LRS-600-36 (Autodesk Fusion 360 design; units mm, degrees)
Autodesk Fusion 360 part; units mm, degrees
sketch "Sketch1" plane through (0, 0, 0) normal (0, 0, 1) x (1, 0, 0)
  line L0 (62, 112.5) -> (-62, 112.5)
  line L1 (-62, 112.5) -> (-62, -112.5)
  line L2 (-62, -112.5) -> (62, -112.5)
  line L3 (62, -112.5) -> (62, 112.5)
  line L4 (62, 112.5) -> (-62, -112.5) construction
  line L5 (-62, 112.5) -> (62, -112.5) construction
  dimension "d1" = 124
  dimension "d2" = 225
  constraint horizontal L0
  constraint perpendicular L0 L1
  constraint parallel L0 L2
  constraint parallel L1 L3
  constraint coincident L4 origin
  constraint coincident L5 origin
  measures "d1" distance of L1.end L2.end
  measures "d2" distance of L0.end L1.end
extrude "Extrude1" add sketch "Sketch1" along normal blind 41 makes body 1
sketch "Sketch2" plane through (62, 0, 0) normal (1, 0, 0) x (0, 1, 0)
  line L0 (-112.5, 0) -> (112.5, 0)
  line L1 (112.5, 0) -> (112.5, 41)
  line L2 (112.5, 41) -> (-112.5, 41)
  line L3 (-112.5, 41) -> (-112.5, 0)
  circle A0 centre (-85.8, 31) radius 2
  circle A1 centre (-85.8, 13) radius 2
  circle A2 centre (74.2, 31) radius 2
  circle A3 centre (74.2, 13) radius 2
  line L4 (-85.8, 0) -> (-85.8, 41) construction
  line L5 (74.2, 0) -> (74.2, 41) construction
  line L6 (-85.8, 31) -> (74.2, 31) construction
  line L7 (-85.8, 13) -> (74.2, 13) construction
  dimension "d5" = 4
  dimension "d6" = 26.7
  dimension "d7" = 160
  dimension "d8" = 13
  dimension "d9" = 18
  constraint equal A0 A1
  constraint equal A1 A2
  constraint equal A2 A3
  constraint coincident L0 L4.start
  constraint coincident L2 L4.end
  constraint perpendicular L2 L4
  constraint coincident L0 L5.start
  constraint coincident L2 L5.end
  constraint perpendicular L2 L5
  constraint coincident A0.centre L4
  constraint coincident A1.centre L4
  constraint coincident A2.centre L5
  constraint coincident A3.centre L5
  constraint coincident A0.centre L6.start
  constraint coincident L5 A2.centre
  constraint perpendicular L5 L6
  constraint coincident A1.centre L7.start
  constraint coincident L5 A3.centre
  constraint perpendicular L5 L7
  constraint coincident A2.centre L6
  constraint coincident A3.centre L7
  measures "d5" diameter of A0
  measures "d6" distance of L3 L4
  measures "d7" distance of L4 L5
  measures "d8" distance of A1.centre L4.start
  measures "d9" distance of A0.centre A1.centre
shell "Shell1" thickness 2 removed faces 0 bodies 1
extrude "Extrude2" cut sketch "Sketch2" against normal through all contours A0 | A1 | A2 | A3 bodies 1
sketch "Sketch3" plane through (0, 0, 41) normal (0, 0, 1) x (-1, 0, 0)
  line L0 (-62, 112.5) -> (-62, -112.5)
  line L1 (-62, -112.5) -> (62, -112.5)
  line L2 (62, -112.5) -> (62, 112.5)
  line L3 (62, 112.5) -> (-62, 112.5)
  line L4 (62, 96.1) -> (-62, 96.1)
  line L5 (-60, 112.5) -> (-60, 96.1)
  line L6 (60, 96.1) -> (60, 112.5)
  dimension "d12" = 16.4
  constraint coincident L2 L4.start
  constraint coincident L0 L4.end
  constraint perpendicular L0 L4
  constraint coincident L4 L6.start
  constraint coincident L4 L5.end
  measures "d12" distance of L3 L4
extrude "Extrude3" cut sketch "Sketch3" against normal up to surface (39 mm away) contours L3 L4 L5 L6 bodies 1
sketch "Sketch4" plane through (0, 0, 0) normal (0, 0, -1) x (1, 0, 0)
  line L0 (62, -112.5) -> (62, 112.5)
  line L1 (62, 112.5) -> (-62, 112.5)
  line L2 (-62, 112.5) -> (-62, -112.5)
  line L3 (-62, -112.5) -> (62, -112.5)
  line L4 (25.5, 79) -> (-24.5, 79) construction
  line L5 (-24.5, 79) -> (-24.5, -71) construction
  line L6 (-24.5, -71) -> (25.5, -71) construction
  line L7 (25.5, -71) -> (25.5, 79) construction
  circle A0 centre (-24.5, 79) radius 2
  circle A1 centre (25.5, 79) radius 2
  circle A2 centre (25.5, -71) radius 2
  circle A3 centre (-24.5, -71) radius 2
  dimension "d18" = 150
  dimension "d19" = 50
  dimension "d21" = 33.5
  dimension "d22" = 37.5
  dimension "d23" = 4
  constraint horizontal L4
  constraint vertical L5
  constraint horizontal L6
  constraint vertical L7
  constraint coincident L4.end L5.start
  constraint coincident L4.start L7.end
  constraint coincident L6.end L7.start
  constraint coincident L5.end L6.start
  constraint equal A0 A1
  constraint equal A1 A2
  constraint equal A2 A3
  measures "d18" distance of L4.start L6.end
  measures "d19" distance of L4.start L4.end
  measures "d21" distance of L1 L4
  measures "d22" distance of L2 L5
  measures "d23" diameter of A0
extrude "Extrude4" cut sketch "Sketch4" against normal blind 2 contours A0 | A1 | A2 | A3 bodies 1
sketch "Sketch5" plane through (0, 0, 2) normal (0, 0, 1) x (-1, 0, 0)
  circle A0 centre (24.5, 79) radius 2
  circle A1 centre (-25.5, -71) radius 2
  circle A2 centre (-25.5, 79) radius 2
  circle A3 centre (24.5, -71) radius 2
  line L0 (-60, 112.5) -> (-60, -110.5)
  line L1 (-60, -110.5) -> (60, -110.5)
  line L2 (60, -110.5) -> (60, 112.5)
  line L3 (60, 112.5) -> (-60, 112.5)
extrude "Extrude5" add sketch "Sketch5" along normal blind 1.7 from surface at 3 separate body contours A0 | A1 | A2 | A3 | L0 L1 L2 L3 makes body 2
sketch "Sketch6" plane through (0, 0, 6.7) normal (0, 0, 1) x (-1, 0, 0)
  line L0 (60, 112.5) -> (-60, 112.5)
  line L1 (-60, 112.5) -> (-60, -110.5)
  line L2 (-60, -110.5) -> (60, -110.5)
  line L3 (60, -110.5) -> (60, 112.5)
  line L4 (-52.7, 110.9) -> (34.3, 110.9)
  line L5 (34.3, 110.9) -> (34.3, 92.9)
  line L6 (34.3, 92.9) -> (-52.7, 92.9)
  line L7 (-52.7, 92.9) -> (-52.7, 110.9)
  dimension "d29" = 87
  dimension "d30" = 18
  dimension "d31" = 1.6
  dimension "d32" = 7.3
  constraint horizontal L4
  constraint vertical L5
  constraint horizontal L6
  constraint vertical L7
  measures "d29" distance of L4.start L4.end
  measures "d30" distance of L4.start L6.end
  measures "d31" distance of L0 L4
  measures "d32" distance of L1 L7
extrude "Extrude6" add sketch "Sketch6" along normal blind 15.4 separate body contours L4 L5 L6 L7 makes body 3
sketch "Sketch7" plane through (0, 0, 6.7) normal (0, 0, 1) x (-1, 0, 0)
  line L0 (60, 112.5) -> (-60, 112.5)
  line L1 (-60, 112.5) -> (-60, -110.5)
  line L2 (-60, -110.5) -> (60, -110.5)
  line L3 (60, -110.5) -> (60, 112.5)
  circle A0 centre (44, 106) radius 3.5
  circle A1 centre (53.5, 107) radius 1.5
  dimension "d35" = 3
  dimension "d36" = 7
  dimension "d37" = 6.5
  dimension "d38" = 5.5
  dimension "d39" = 6.5
  dimension "d40" = 16
  measures "d35" diameter of A1
  measures "d36" diameter of A0
  measures "d37" distance of L3 A1.centre
  measures "d38" distance of L0 A1.centre
  measures "d39" distance of L0 A0.centre
  measures "d40" distance of L3 A0.centre
extrude "Extrude7" add sketch "Sketch7" along normal blind 10 contours A1 bodies 2
extrude "Extrude8" add sketch "Sketch7" along normal blind 8 contours A0 bodies 2
sketch "Sketch8" plane through (0, 0, 22.1) normal (0, 0, 1) x (-1, 0, 0)
  line L0 (-52.7, 92.9) -> (34.3, 92.9)
  line L1 (34.3, 92.9) -> (34.3, 110.9)
  line L2 (34.3, 110.9) -> (-52.7, 110.9)
  line L3 (-52.7, 110.9) -> (-52.7, 92.9)
  line L4 (-52.7, 110.9) -> (-51.5, 110.9)
  line L5 (-51.5, 110.9) -> (-51.5, 95.9)
  line L6 (-51.5, 95.9) -> (-43.3, 95.9)
  line L7 (-43.3, 95.9) -> (-43.3, 110.9)
  line L8 (-41.95, 110.9) -> (-41.95, 95.9)
  line L9 (-41.95, 95.9) -> (-33.75, 95.9)
  line L10 (-33.75, 95.9) -> (-33.75, 110.9)
  line L11 (-32.4, 110.9) -> (-32.4, 95.9)
  line L12 (-32.4, 95.9) -> (-24.2, 95.9)
  line L13 (-24.2, 95.9) -> (-24.2, 110.9)
  line L14 (-22.85, 110.9) -> (-22.85, 95.9)
  line L15 (-22.85, 95.9) -> (-14.65, 95.9)
  line L16 (-14.65, 95.9) -> (-14.65, 110.9)
  line L17 (-13.3, 110.9) -> (-13.3, 95.9)
  line L18 (-13.3, 95.9) -> (-5.1, 95.9)
  line L19 (-5.1, 95.9) -> (-5.1, 110.9)
  line L20 (-3.75, 110.9) -> (-3.75, 95.9)
  line L21 (-3.75, 95.9) -> (4.45, 95.9)
  line L22 (4.45, 95.9) -> (4.45, 110.9)
  line L23 (5.8, 110.9) -> (5.8, 95.9)
  line L24 (5.8, 95.9) -> (14, 95.9)
  line L25 (14, 95.9) -> (14, 110.9)
  line L26 (15.35, 110.9) -> (15.35, 95.9)
  line L27 (15.35, 95.9) -> (23.55, 95.9)
  line L28 (23.55, 95.9) -> (23.55, 110.9)
  line L29 (24.9, 110.9) -> (24.9, 95.9)
  line L30 (24.9, 95.9) -> (33.1, 95.9)
  line L31 (33.1, 95.9) -> (33.1, 110.9)
  line L32 (24.9, 110.9) -> (23.55, 110.9)
  line L33 (15.35, 110.9) -> (14, 110.9)
  line L34 (5.8, 110.9) -> (4.45, 110.9)
  line L35 (-3.75, 110.9) -> (-5.1, 110.9)
  line L36 (-13.3, 110.9) -> (-14.65, 110.9)
  line L37 (-22.85, 110.9) -> (-24.2, 110.9)
  line L38 (-32.4, 110.9) -> (-33.75, 110.9)
  line L39 (-41.95, 110.9) -> (-43.3, 110.9)
  line L40 (34.3, 110.9) -> (33.1, 110.9)
  dimension "d45" = 8.2
  dimension "d46" = 1.35
  dimension "d47" = 15
  constraint coincident L2.end L3.start
  constraint coincident L2 L4.end
  constraint perpendicular L3 L4
  constraint perpendicular L4 L5
  constraint perpendicular L3 L6
  constraint coincident L2 L7.end
  constraint perpendicular L4 L7
  constraint perpendicular L4 L8
  constraint perpendicular L7 L9
  constraint coincident L2 L10.end
  constraint perpendicular L2 L10
  constraint coincident L2 L11.start
  constraint perpendicular L2 L11
  constraint perpendicular L11 L12
  constraint coincident L2 L13.end
  constraint perpendicular L2 L13
  constraint coincident L2 L14.start
  constraint perpendicular L2 L14
  constraint perpendicular L14 L15
  constraint coincident L2 L16.end
  constraint perpendicular L2 L16
  constraint coincident L2 L17.start
  constraint perpendicular L2 L17
  constraint perpendicular L17 L18
  constraint coincident L2 L19.end
  constraint perpendicular L2 L19
  constraint coincident L2 L20.start
  constraint perpendicular L2 L20
  constraint perpendicular L19 L21
  constraint coincident L2 L22.end
  constraint perpendicular L21 L22
  constraint coincident L2 L23.start
  constraint perpendicular L2 L23
  constraint perpendicular L19 L24
  constraint coincident L2 L25.end
  constraint perpendicular L2 L25
  constraint coincident L2 L26.start
  constraint perpendicular L2 L26
  constraint perpendicular L26 L27
  constraint coincident L2 L28.end
  constraint perpendicular L2 L28
  constraint coincident L2 L29.start
  constraint perpendicular L2 L29
  constraint perpendicular L29 L30
  constraint coincident L2 L31.end
  constraint perpendicular L2 L31
  constraint equal L27 L30
  constraint equal L24 L27
  constraint equal L21 L24
  constraint equal L18 L21
  constraint equal L15 L18
  constraint equal L12 L15
  constraint equal L9 L12
  constraint equal L6 L9
  constraint perpendicular L8 L39
  constraint equal L38 L39
  constraint equal L37 L38
  constraint equal L36 L37
  constraint equal L35 L36
  constraint equal L34 L35
  constraint equal L33 L34
  constraint equal L32 L33
  constraint coincident L1.end L2.start
  constraint equal L4 L40
  constraint collinear L27 L30
  constraint collinear L24 L27
  constraint collinear L21 L24
  constraint collinear L15 L21
  constraint collinear L15 L18
  constraint collinear L12 L18
  constraint collinear L9 L12
  constraint collinear L6 L9
  measures "d45" distance of L29.end L30.end
  measures "d46" distance of L7.end L8.start
  measures "d47" distance of L4.end L5.end
extrude "Extrude9" cut sketch "Sketch8" against normal blind 8 contours L2 L5 L6 L7 | L2 L29 L30 L31 | L2 L8 L9 L10 | L2 L26 L27 L28 | L2 L11 L12 L13 | L2 L23 L24 L25 | L2 L14 L15 L16 | L2 L20 L21 L22 | L2 L17 L18 L19 bodies 3
sketch "Sketch9" plane through (0, 0, 41) normal (0, 0, 1) x (-1, 0, 0)
  line L0 (-60, 96.1) -> (-60, 112.5)
  line L1 (-60, 112.5) -> (-62, 112.5)
  line L2 (-62, 112.5) -> (-62, -112.5)
  line L3 (-62, -112.5) -> (62, -112.5)
  line L4 (62, -112.5) -> (62, 112.5)
  line L5 (62, 112.5) -> (60, 112.5)
  line L6 (60, 112.5) -> (60, 96.1)
  line L7 (60, 96.1) -> (-60, 96.1)
  circle A0 centre (24.5, -62.5) radius 30 construction
  circle A1 centre (24.5, -62.5) radius 26.5 construction
  circle A2 centre (24.5, -62.5) radius 18.5 construction
  circle A3 centre (24.5, -62.5) radius 21.5
  circle A4 centre (24.5, -62.5) radius 15.5
  circle A5 centre (24.5, -62.5) radius 29.5
  circle A6 centre (24.5, -62.5) radius 23.5
  line L8 (24.5, -62.5) -> (62, -62.5) construction
  line L9 (24.5, -62.5) -> (62, -72.5481) construction
  circle A7 centre (42.3696, -67.2882) radius 3
  circle A8 centre (42.3696, -57.7118) radius 3
  circle A9 centre (37.5815, -49.4185) radius 3
  circle A10 centre (29.2882, -44.6304) radius 3
  circle A11 centre (19.7118, -44.6304) radius 3
  circle A12 centre (11.4185, -49.4185) radius 3
  circle A13 centre (6.6304, -57.7118) radius 3
  circle A14 centre (6.6304, -67.2882) radius 3
  circle A15 centre (11.4185, -75.5815) radius 3
  circle A16 centre (19.7118, -80.3696) radius 3
  circle A17 centre (29.2882, -80.3696) radius 3
  circle A18 centre (37.5815, -75.5815) radius 3
  line L10 (24.5, -62.5) -> (25.2686, -62.7059) construction
  line L11 (24.5, -62.5) -> (62, -69.1123) construction
  circle A19 centre (50.5974, -67.1017) radius 3
  circle A20 centre (50.5974, -57.8983) radius 3
  circle A21 centre (47.4497, -49.25) radius 3
  circle A22 centre (41.5339, -42.1998) radius 3
  circle A23 centre (33.5635, -37.5981) radius 3
  circle A24 centre (24.5, -36) radius 3
  circle A25 centre (15.4365, -37.5981) radius 3
  circle A26 centre (7.4661, -42.1998) radius 3
  circle A27 centre (1.5503, -49.25) radius 3
  circle A28 centre (-1.5974, -57.8983) radius 3
  circle A29 centre (-1.5974, -67.1017) radius 3
  circle A30 centre (1.5503, -75.75) radius 3
  circle A31 centre (7.4661, -82.8002) radius 3
  circle A32 centre (15.4365, -87.4019) radius 3
  circle A33 centre (24.5, -89) radius 3
  circle A34 centre (33.5635, -87.4019) radius 3
  circle A35 centre (41.5339, -82.8002) radius 3
  circle A36 centre (47.4497, -75.75) radius 3
  dimension "d50" = 37.5
  dimension "d51" = 50
  dimension "d52" = 60
  dimension "d53" = 53
  dimension "d54" = 37
  dimension "d55" = 3
  dimension "d56" = -3
  dimension "d57" = 3
  dimension "d58" = -3
  dimension "d59" = 15
  dimension "d61" = 360
  dimension "d62" = 10
  dimension "d64" = 360
  constraint concentric A0 A1
  constraint concentric A0 A2
  constraint coincident A0.centre A1.centre
  constraint perpendicular L4 L8
  constraint coincident L4 L9.end
  constraint coincident L4 L8.end
  constraint coincident A2 A7.centre
  constraint coincident L9 A7.centre
  constraint tangent A4 A7
  constraint coincident L9 L10.end
  constraint coincident L4 L11.end
  constraint coincident A1 A19.centre
  constraint coincident L11 A19.centre
  constraint tangent A6 A19
  measures "d50" distance of L4 A0.centre
  measures "d51" distance of L3 A0.centre
  measures "d52" diameter of A0
  measures "d53" diameter of A1
  measures "d54" diameter of A2
  measures "d59" angle of L8 L9
  measures "d62" angle of L8 L11
extrude "Extrude10" cut sketch "Sketch9" against normal blind 2 contours A3 A4 A7 A8 | A8 | A7 | A3 A4 A9 A10 | A9 | A3 A4 A17 A18 | A18 | A10 | A17 | A3 A4 A11 A12 | A11 | A3 A4 A15 A16 | A16 | A12 | A15 | A3 A4 A13 A14 | A13 | A14 | A5 A6 A20 A21 | A20 | A5 A6 A19 A36 | A19 | A5 A6 A21 A22 | A21 | A5 A6 A35 A36 | A36 | A22 | A35 | A5 A6 A23 A24 | A23 | A5 A6 A33 A34 | A34 | A5 A6 A24 A25 | A24 | A5 A6 A32 A33 | A33 | A25 | A32 | A5 A6 A26 A27 | A26 | A5 A6 A30 A31 | A31 | A5 A6 A27 A28 | A27 | A5 A6 A29 A30 | A30 | A28 | A29 bodies 1
sketch "Sketch10" plane through (0, 0, 41) normal (0, 0, 1) x (-1, 0, 0)
  arc A0 (14.4104, -90.2209) -> (34.5896, -90.2209) centre (24.5, -62.5) ccw
  arc A1 (16.4625, -84.5828) -> (14.4104, -90.2209) centre (15.4365, -87.4019) ccw
  arc A2 (16.4625, -84.5828) -> (32.5375, -84.5828) centre (24.5, -62.5) ccw
  arc A3 (34.5896, -90.2209) -> (32.5375, -84.5828) centre (33.5635, -87.4019) ccw
  arc A4 (18.9354, -41.7326) -> (9.2972, -47.2972) centre (24.5, -62.5) ccw
  arc A5 (20.4883, -47.5281) -> (18.9354, -41.7326) centre (19.7118, -44.6304) ccw
  arc A6 (20.4883, -47.5281) -> (13.5398, -51.5398) centre (24.5, -62.5) ccw
  arc A7 (9.2972, -47.2972) -> (13.5398, -51.5398) centre (11.4185, -49.4185) ccw
  arc A8 (45.2674, -68.0646) -> (45.2674, -56.9354) centre (24.5, -62.5) ccw
  arc A9 (39.4719, -66.5117) -> (45.2674, -68.0646) centre (42.3696, -67.2882) ccw
  arc A10 (39.4719, -66.5117) -> (39.4719, -58.4883) centre (24.5, -62.5) ccw
  arc A11 (45.2674, -56.9354) -> (39.4719, -58.4883) centre (42.3696, -57.7118) ccw
  arc A12 (30.0646, -83.2674) -> (39.7028, -77.7028) centre (24.5, -62.5) ccw
  arc A13 (28.5117, -77.4719) -> (30.0646, -83.2674) centre (29.2882, -80.3696) ccw
  arc A14 (28.5117, -77.4719) -> (35.4602, -73.4602) centre (24.5, -62.5) ccw
  arc A15 (39.7028, -77.7028) -> (35.4602, -73.4602) centre (37.5815, -75.5815) ccw
  arc A16 (34.5896, -34.7791) -> (14.4104, -34.7791) centre (24.5, -62.5) ccw
  arc A17 (32.5375, -40.4172) -> (34.5896, -34.7791) centre (33.5635, -37.5981) ccw
  arc A18 (32.5375, -40.4172) -> (16.4625, -40.4172) centre (24.5, -62.5) ccw
  arc A19 (14.4104, -34.7791) -> (16.4625, -40.4172) centre (15.4365, -37.5981) ccw
  arc A20 (43.4622, -85.0983) -> (53.5518, -67.6226) centre (24.5, -62.5) ccw
  arc A21 (39.6055, -80.502) -> (43.4622, -85.0983) centre (41.5339, -82.8002) ccw
  arc A22 (39.6055, -80.502) -> (47.643, -66.5807) centre (24.5, -62.5) ccw
  arc A23 (53.5518, -67.6226) -> (47.643, -66.5807) centre (50.5974, -67.1017) ccw
  arc A24 (-4.5518, -67.6226) -> (5.5378, -85.0983) centre (24.5, -62.5) ccw
  arc A25 (1.357, -66.5807) -> (-4.5518, -67.6226) centre (-1.5974, -67.1017) ccw
  arc A26 (1.357, -66.5807) -> (9.3945, -80.502) centre (24.5, -62.5) ccw
  arc A27 (5.5378, -85.0983) -> (9.3945, -80.502) centre (7.4661, -82.8002) ccw
  arc A28 (3.7326, -56.9354) -> (3.7326, -68.0646) centre (24.5, -62.5) ccw
  arc A29 (9.5281, -58.4883) -> (3.7326, -56.9354) centre (6.6304, -57.7118) ccw
  arc A30 (9.5281, -58.4883) -> (9.5281, -66.5117) centre (24.5, -62.5) ccw
  arc A31 (3.7326, -68.0646) -> (9.5281, -66.5117) centre (6.6304, -67.2882) ccw
  arc A32 (39.7028, -47.2972) -> (30.0646, -41.7326) centre (24.5, -62.5) ccw
  arc A33 (35.4602, -51.5398) -> (39.7028, -47.2972) centre (37.5815, -49.4185) ccw
  arc A34 (35.4602, -51.5398) -> (28.5117, -47.5281) centre (24.5, -62.5) ccw
  arc A35 (30.0646, -41.7326) -> (28.5117, -47.5281) centre (29.2882, -44.6304) ccw
  arc A36 (9.2972, -77.7028) -> (18.9354, -83.2674) centre (24.5, -62.5) ccw
  arc A37 (13.5398, -73.4602) -> (9.2972, -77.7028) centre (11.4185, -75.5815) ccw
  arc A38 (13.5398, -73.4602) -> (20.4883, -77.4719) centre (24.5, -62.5) ccw
  arc A39 (18.9354, -83.2674) -> (20.4883, -77.4719) centre (19.7118, -80.3696) ccw
  arc A40 (5.5378, -39.9017) -> (-4.5518, -57.3774) centre (24.5, -62.5) ccw
  arc A41 (9.3945, -44.498) -> (5.5378, -39.9017) centre (7.4661, -42.1998) ccw
  arc A42 (9.3945, -44.498) -> (1.357, -58.4193) centre (24.5, -62.5) ccw
  arc A43 (-4.5518, -57.3774) -> (1.357, -58.4193) centre (-1.5974, -57.8983) ccw
  arc A44 (53.5518, -57.3774) -> (43.4622, -39.9017) centre (24.5, -62.5) ccw
  arc A45 (47.643, -58.4193) -> (53.5518, -57.3774) centre (50.5974, -57.8983) ccw
  arc A46 (47.643, -58.4193) -> (39.6055, -44.498) centre (24.5, -62.5) ccw
  arc A47 (43.4622, -39.9017) -> (39.6055, -44.498) centre (41.5339, -42.1998) ccw
  line L0 (-60, 96.1) -> (-60, 112.5)
  line L1 (-60, 112.5) -> (-62, 112.5)
  line L2 (-62, 112.5) -> (-62, -112.5)
  line L3 (-62, -112.5) -> (62, -112.5)
  line L4 (62, -112.5) -> (62, 112.5)
  line L5 (62, 112.5) -> (60, 112.5)
  line L6 (60, 112.5) -> (60, 96.1)
  line L7 (60, 96.1) -> (-60, 96.1)
  circle A48 centre (24.5, -62.5) radius 30
  line L8 (20, -67) -> (29, -67) construction
  line L9 (29, -67) -> (29, -58) construction
  line L10 (29, -58) -> (20, -58) construction
  line L11 (20, -58) -> (20, -67) construction
  line L12 (20, -67) -> (29, -58) construction
  line L13 (29, -67) -> (20, -58) construction
  circle A49 centre (29, -67) radius 2
  circle A50 centre (20, -67) radius 2
  circle A51 centre (20, -58) radius 2
  circle A52 centre (29, -58) radius 2
  point P0 (24.5, -62.5)
  point P1 (24.5, -62.5)
  dimension "d67" = 9
  dimension "d68" = 4
  constraint horizontal L8
  constraint perpendicular L8 L9
  constraint parallel L8 L10
  constraint parallel L9 L11
  constraint coincident L12 P1
  constraint coincident L13 P1
  constraint coincident P1 P0
  constraint equal L8 L11
  constraint coincident L8.end L9.start
  constraint coincident L8.start L11.end
  constraint coincident L10.end L11.start
  constraint coincident L9.end L10.start
  constraint equal A49 A52
  constraint equal A49 A50
  constraint equal A50 A51
  measures "d67" distance of L8.start L8.end
  measures "d68" diameter of A51
extrude "Extrude11" cut sketch "Sketch10" against normal blind 2 contours A49 | A50 | A51 | A52 bodies 1
sketch "Sketch11" plane through (0, 0, 41) normal (0, 0, 1) x (-1, 0, 0)
  circle A0 centre (29, -58) radius 2
  circle A1 centre (29, -67) radius 2
  circle A2 centre (20, -58) radius 2
  circle A3 centre (20, -67) radius 2
  arc A4 (14.4104, -90.2209) -> (34.5896, -90.2209) centre (24.5, -62.5) ccw
  arc A5 (16.4625, -84.5828) -> (14.4104, -90.2209) centre (15.4365, -87.4019) ccw
  arc A6 (16.4625, -84.5828) -> (32.5375, -84.5828) centre (24.5, -62.5) ccw
  arc A7 (34.5896, -90.2209) -> (32.5375, -84.5828) centre (33.5635, -87.4019) ccw
  arc A8 (18.9354, -41.7326) -> (9.2972, -47.2972) centre (24.5, -62.5) ccw
  arc A9 (20.4883, -47.5281) -> (18.9354, -41.7326) centre (19.7118, -44.6304) ccw
  arc A10 (20.4883, -47.5281) -> (13.5398, -51.5398) centre (24.5, -62.5) ccw
  arc A11 (9.2972, -47.2972) -> (13.5398, -51.5398) centre (11.4185, -49.4185) ccw
  arc A12 (45.2674, -68.0646) -> (45.2674, -56.9354) centre (24.5, -62.5) ccw
  arc A13 (39.4719, -66.5117) -> (45.2674, -68.0646) centre (42.3696, -67.2882) ccw
  arc A14 (39.4719, -66.5117) -> (39.4719, -58.4883) centre (24.5, -62.5) ccw
  arc A15 (45.2674, -56.9354) -> (39.4719, -58.4883) centre (42.3696, -57.7118) ccw
  arc A16 (30.0646, -83.2674) -> (39.7028, -77.7028) centre (24.5, -62.5) ccw
  arc A17 (28.5117, -77.4719) -> (30.0646, -83.2674) centre (29.2882, -80.3696) ccw
  arc A18 (28.5117, -77.4719) -> (35.4602, -73.4602) centre (24.5, -62.5) ccw
  arc A19 (39.7028, -77.7028) -> (35.4602, -73.4602) centre (37.5815, -75.5815) ccw
  arc A20 (34.5896, -34.7791) -> (14.4104, -34.7791) centre (24.5, -62.5) ccw
  arc A21 (32.5375, -40.4172) -> (34.5896, -34.7791) centre (33.5635, -37.5981) ccw
  arc A22 (32.5375, -40.4172) -> (16.4625, -40.4172) centre (24.5, -62.5) ccw
  arc A23 (14.4104, -34.7791) -> (16.4625, -40.4172) centre (15.4365, -37.5981) ccw
  arc A24 (43.4622, -85.0983) -> (53.5518, -67.6226) centre (24.5, -62.5) ccw
  arc A25 (39.6055, -80.502) -> (43.4622, -85.0983) centre (41.5339, -82.8002) ccw
  arc A26 (39.6055, -80.502) -> (47.643, -66.5807) centre (24.5, -62.5) ccw
  arc A27 (53.5518, -67.6226) -> (47.643, -66.5807) centre (50.5974, -67.1017) ccw
  arc A28 (-4.5518, -67.6226) -> (5.5378, -85.0983) centre (24.5, -62.5) ccw
  arc A29 (1.357, -66.5807) -> (-4.5518, -67.6226) centre (-1.5974, -67.1017) ccw
  arc A30 (1.357, -66.5807) -> (9.3945, -80.502) centre (24.5, -62.5) ccw
  arc A31 (5.5378, -85.0983) -> (9.3945, -80.502) centre (7.4661, -82.8002) ccw
  arc A32 (3.7326, -56.9354) -> (3.7326, -68.0646) centre (24.5, -62.5) ccw
  arc A33 (9.5281, -58.4883) -> (3.7326, -56.9354) centre (6.6304, -57.7118) ccw
  arc A34 (9.5281, -58.4883) -> (9.5281, -66.5117) centre (24.5, -62.5) ccw
  arc A35 (3.7326, -68.0646) -> (9.5281, -66.5117) centre (6.6304, -67.2882) ccw
  arc A36 (39.7028, -47.2972) -> (30.0646, -41.7326) centre (24.5, -62.5) ccw
  arc A37 (35.4602, -51.5398) -> (39.7028, -47.2972) centre (37.5815, -49.4185) ccw
  arc A38 (35.4602, -51.5398) -> (28.5117, -47.5281) centre (24.5, -62.5) ccw
  arc A39 (30.0646, -41.7326) -> (28.5117, -47.5281) centre (29.2882, -44.6304) ccw
  arc A40 (9.2972, -77.7028) -> (18.9354, -83.2674) centre (24.5, -62.5) ccw
  arc A41 (13.5398, -73.4602) -> (9.2972, -77.7028) centre (11.4185, -75.5815) ccw
  arc A42 (13.5398, -73.4602) -> (20.4883, -77.4719) centre (24.5, -62.5) ccw
  arc A43 (18.9354, -83.2674) -> (20.4883, -77.4719) centre (19.7118, -80.3696) ccw
  arc A44 (5.5378, -39.9017) -> (-4.5518, -57.3774) centre (24.5, -62.5) ccw
  arc A45 (9.3945, -44.498) -> (5.5378, -39.9017) centre (7.4661, -42.1998) ccw
  arc A46 (9.3945, -44.498) -> (1.357, -58.4193) centre (24.5, -62.5) ccw
  arc A47 (-4.5518, -57.3774) -> (1.357, -58.4193) centre (-1.5974, -57.8983) ccw
  arc A48 (53.5518, -57.3774) -> (43.4622, -39.9017) centre (24.5, -62.5) ccw
  arc A49 (47.643, -58.4193) -> (53.5518, -57.3774) centre (50.5974, -57.8983) ccw
  arc A50 (47.643, -58.4193) -> (39.6055, -44.498) centre (24.5, -62.5) ccw
  arc A51 (43.4622, -39.9017) -> (39.6055, -44.498) centre (41.5339, -42.1998) ccw
  line L0 (-60, 96.1) -> (-60, 112.5)
  line L1 (-60, 112.5) -> (-62, 112.5)
  line L2 (-62, 112.5) -> (-62, -112.5)
  line L3 (-62, -112.5) -> (62, -112.5)
  line L4 (62, -112.5) -> (62, 112.5)
  line L5 (62, 112.5) -> (60, 112.5)
  line L6 (60, 112.5) -> (60, 96.1)
  line L7 (60, 96.1) -> (-60, 96.1)
  line L8 (62, 41.8) -> (-62, 41.8) construction
  line L9 (42.3, 41.8) -> (42.3, 39.3) construction
  line L10 (12.3, 41.8) -> (12.3, 39.3) construction
  line L11 (42.3, 41.8) -> (42.3, 44.3) construction
  line L12 (12.3, 41.8) -> (12.3, 44.3) construction
  line L13 (42.3, 39.3) -> (12.3, 39.3)
  line L14 (12.3, 44.3) -> (42.3, 44.3)
  arc A52 (42.3, 39.3) -> (42.3, 44.3) centre (42.3, 41.8) ccw
  arc A53 (12.3, 44.3) -> (12.3, 39.3) centre (12.3, 41.8) ccw
  line L15 (42.3, 41.8) -> (42.3, 15.1224) construction
  line L16 (42.3, 41.8) -> (42.3, 79.2423) construction
  line L17 (42.3, 29.3) -> (12.3, 29.3)
  arc A54 (42.3, 29.3) -> (42.3, 34.3) centre (42.3, 31.8) ccw
  line L18 (12.3, 34.3) -> (42.3, 34.3)
  arc A55 (12.3, 34.3) -> (12.3, 29.3) centre (12.3, 31.8) ccw
  line L19 (42.3, 19.3) -> (12.3, 19.3)
  arc A56 (42.3, 19.3) -> (42.3, 24.3) centre (42.3, 21.8) ccw
  line L20 (12.3, 24.3) -> (42.3, 24.3)
  arc A57 (12.3, 24.3) -> (12.3, 19.3) centre (12.3, 21.8) ccw
  line L21 (12.3, 74.3) -> (42.3, 74.3)
  arc A58 (42.3, 69.3) -> (42.3, 74.3) centre (42.3, 71.8) ccw
  line L22 (42.3, 69.3) -> (12.3, 69.3)
  arc A59 (12.3, 74.3) -> (12.3, 69.3) centre (12.3, 71.8) ccw
  arc A60 (-45.7, 34.3) -> (-45.7, 29.3) centre (-45.7, 31.8) ccw
  line L23 (-45.7, 34.3) -> (-15.7, 34.3)
  arc A61 (-15.7, 29.3) -> (-15.7, 34.3) centre (-15.7, 31.8) ccw
  line L24 (-15.7, 29.3) -> (-45.7, 29.3)
  dimension "d71" = 5
  dimension "d72" = 30
  dimension "d73" = 19.7
  dimension "d76" = 0
  dimension "d77" = -10
  dimension "d80" = 0
  dimension "d81" = 30
  dimension "d82" = 21.8
  dimension "d85" = -58
  dimension "d86" = 0
  constraint coincident L4 L8.start
  constraint coincident L2 L8.end
  constraint perpendicular L2 L8
  constraint coincident L8 L9.start
  constraint coincident L8 L10.start
  constraint equal A52 A53
  constraint coincident L9.start L11.start
  constraint perpendicular L8 L9
  constraint coincident L10.start L12.start
  constraint perpendicular L8 L10
  constraint parallel L10 L11
  constraint perpendicular L8 L12
  constraint tangent L14 A53
  constraint perpendicular L13 L15
  constraint perpendicular L14 L16
  measures "d71" diameter of A53
  measures "d72" distance of L9.start L10.start
  measures "d73" distance of L4 L9.start
  measures "d82" distance of L7 L21
extrude "Extrude12" cut sketch "Sketch11" against normal blind 2 contours L13 L14 A52 A53 | L17 A54 L18 A55 | L19 A56 L20 A57 | L21 A58 L22 A59 | A60 L23 A61 L24 bodies 1
sketch "Sketch12" plane through (62, 0, 0) normal (1, 0, 0) x (0, 1, 0)
  circle A0 centre (-85.8, 13) radius 2
  circle A1 centre (74.2, 31) radius 2
  circle A2 centre (-85.8, 31) radius 2
  circle A3 centre (74.2, 13) radius 2
  line L0 (-112.5, 0) -> (112.5, 0)
  line L1 (112.5, 0) -> (112.5, 41)
  line L2 (112.5, 41) -> (-112.5, 41)
  line L3 (-112.5, 41) -> (-112.5, 0)
  line L4 (-93.5, 20.2) -> (-91, 20.2)
  line L5 (-91, 20.2) -> (-91, 13.3)
  line L6 (-91, 13.3) -> (-93.5, 13.3)
  line L7 (-93.5, 13.3) -> (-93.5, 20.2)
  line L8 (-81.4787, 20.2) -> (-78.9787, 20.2)
  line L9 (-78.9787, 20.2) -> (-78.9787, 13.3)
  line L10 (-78.9787, 13.3) -> (-81.4787, 13.3)
  line L11 (-81.4787, 13.3) -> (-81.4787, 20.2)
  line L12 (-85.8, 13) -> (-85.8, 31) construction
  line L13 (74.2, 31) -> (74.2, 13) construction
  line L14 (81.9, 20.2) -> (81.9, 13.3)
  line L15 (79.4, 13.3) -> (79.4, 20.2)
  line L16 (69, 20.2) -> (69, 13.3)
  line L17 (79.4, 20.2) -> (81.9, 20.2)
  line L18 (69, 13.3) -> (66.5, 13.3)
  line L19 (81.9, 13.3) -> (79.4, 13.3)
  line L20 (66.5, 13.3) -> (66.5, 20.2)
  line L21 (66.5, 20.2) -> (69, 20.2)
  point P0 (73.9672, 16.2288)
  point P1 (73.9672, 16.2288)
  dimension "d89" = 2.5
  dimension "d90" = 6.9
  dimension "d91" = 5.2
  dimension "d92" = 4.3213
  dimension "d93" = 13.3
  dimension "d94" = 2.5
  dimension "d95" = 6.9
  dimension "d96" = 5.2
  dimension "d97" = 13.3
  dimension "d98" = 5.2
  constraint horizontal L4
  constraint vertical L5
  constraint horizontal L6
  constraint vertical L7
  constraint horizontal L8
  constraint vertical L9
  constraint horizontal L10
  constraint vertical L11
  constraint equal L4 L8
  constraint equal L7 L11
  constraint collinear L4 L8
  constraint coincident A0.centre L12.start
  constraint coincident A2.centre L12.end
  constraint coincident A1.centre L13.start
  constraint coincident A3.centre L13.end
  constraint horizontal L21
  constraint vertical L16
  constraint horizontal L18
  constraint vertical L20
  constraint horizontal L17
  constraint vertical L14
  constraint horizontal L19
  constraint vertical L15
  constraint equal L17 L21
  constraint equal L15 L20
  constraint collinear L17 L21
  constraint coincident P1 P0
  measures "d89" distance of L5.end L6.end
  measures "d90" distance of L4.start L6.end
  measures "d91" distance of L5 L12
  measures "d92" distance of L11 L12
  measures "d93" distance of L0 L6
  measures "d94" distance of L18.end L16.end
  measures "d95" distance of L20.end L18.end
  measures "d96" distance of L13 L16
  measures "d97" distance of L0 L18
  measures "d98" distance of L13 L15
extrude "Extrude13" cut sketch "Sketch12" against normal through all contours L4 L5 L6 L7 | L8 L9 L10 L11 | L14 L15 L17 L19 | L16 L18 L20 L21 bodies 1
sketch "Sketch13" plane through (62, 0, 0) normal (1, 0, 0) x (0, 1, 0)
  line L0 (66.5, 20.2) -> (69, 20.2)
  line L1 (69, 20.2) -> (69, 13.3)
  line L2 (69, 13.3) -> (66.5, 13.3)
  line L3 (66.5, 13.3) -> (66.5, 20.2)
  line L4 (-93.5, 13.3) -> (-93.5, 20.2)
  line L5 (-93.5, 20.2) -> (-91, 20.2)
  line L6 (-91, 20.2) -> (-91, 13.3)
  line L7 (-91, 13.3) -> (-93.5, 13.3)
  line L8 (81.9, 13.3) -> (79.4, 13.3)
  line L9 (79.4, 13.3) -> (79.4, 20.2)
  line L10 (79.4, 20.2) -> (81.9, 20.2)
  line L11 (81.9, 20.2) -> (81.9, 13.3)
  line L12 (-81.4787, 13.3) -> (-81.4787, 20.2)
  line L13 (-81.4787, 20.2) -> (-78.9787, 20.2)
  line L14 (-78.9787, 20.2) -> (-78.9787, 13.3)
  line L15 (-78.9787, 13.3) -> (-81.4787, 13.3)
  circle A0 centre (-85.8, 13) radius 2
  circle A1 centre (74.2, 31) radius 2
  circle A2 centre (-85.8, 31) radius 2
  circle A3 centre (74.2, 13) radius 2
  line L16 (-112.5, 0) -> (112.5, 0)
  line L17 (112.5, 0) -> (112.5, 41)
  line L18 (112.5, 41) -> (-112.5, 41)
  line L19 (-112.5, 41) -> (-112.5, 0)
  line L20 (47, 17.6) -> (62, 17.6)
  line L21 (62, 17.6) -> (62, 8.6)
  line L22 (62, 8.6) -> (47, 8.6)
  line L23 (47, 8.6) -> (47, 17.6)
  dimension "d100" = 15
  dimension "d101" = 9
  dimension "d102" = 8.6
  dimension "d103" = 50.5
  constraint horizontal L20
  constraint vertical L21
  constraint horizontal L22
  constraint vertical L23
  measures "d100" distance of L20.start L20.end
  measures "d101" distance of L20.start L22.end
  measures "d102" distance of L16 L22
  measures "d103" distance of L17 L21
extrude "Extrude14" cut sketch "Sketch13" against normal blind 2 contours L20 L21 L22 L23 bodies 1
sketch "Sketch14" plane through (62, 0, 0) normal (1, 0, 0) x (0, 1, 0)
  line L0 (62, 17.6) -> (62, 8.6)
  line L1 (62, 8.6) -> (47, 8.6)
  line L2 (47, 8.6) -> (47, 17.6)
  line L3 (47, 17.6) -> (62, 17.6)
  line L4 (66.5, 20.2) -> (69, 20.2)
  line L5 (69, 20.2) -> (69, 13.3)
  line L6 (69, 13.3) -> (66.5, 13.3)
  line L7 (66.5, 13.3) -> (66.5, 20.2)
  line L8 (-93.5, 13.3) -> (-93.5, 20.2)
  line L9 (-93.5, 20.2) -> (-91, 20.2)
  line L10 (-91, 20.2) -> (-91, 13.3)
  line L11 (-91, 13.3) -> (-93.5, 13.3)
  line L12 (81.9, 13.3) -> (79.4, 13.3)
  line L13 (79.4, 13.3) -> (79.4, 20.2)
  line L14 (79.4, 20.2) -> (81.9, 20.2)
  line L15 (81.9, 20.2) -> (81.9, 13.3)
  line L16 (-81.4787, 13.3) -> (-81.4787, 20.2)
  line L17 (-81.4787, 20.2) -> (-78.9787, 20.2)
  line L18 (-78.9787, 20.2) -> (-78.9787, 13.3)
  line L19 (-78.9787, 13.3) -> (-81.4787, 13.3)
  circle A0 centre (-85.8, 13) radius 2
  circle A1 centre (74.2, 31) radius 2
  circle A2 centre (-85.8, 31) radius 2
  circle A3 centre (74.2, 13) radius 2
  line L20 (-112.5, 0) -> (112.5, 0)
  line L21 (112.5, 0) -> (112.5, 41)
  line L22 (112.5, 41) -> (-112.5, 41)
  line L23 (-112.5, 41) -> (-112.5, 0)
  line L24 (-112.5, 5) -> (110.5, 5)
  line L25 (43.4, 5) -> (43.4, 21.2)
  line L26 (43.4, 21.2) -> (65.6, 21.2)
  line L27 (65.6, 21.2) -> (65.6, 5)
  line L28 (65.6, 5) -> (43.4, 5)
  dimension "d106" = -3.6
extrude "Extrude15" add sketch "Sketch14" against normal blind 7 from surface at -5 separate body contours L24 L25 L26 L27 L28 makes body 4
extrude "Extrude16" add sketch "Sketch14" along normal blind 6.9 from surface at -12 contours L0 L1 L2 L3 bodies 4
extrude "Extrude17" cut 1 faces at (54.6667, 50.8, 5) along direction (0, 0, 1) blind 1.7 on bodies 4 bodies 4
sketch "Sketch15" plane through (0, 0, 39) normal (0, 0, -1) x (1, 0, 0)
  line L0 (-42.3, 34.3) -> (-12.3, 34.3)
  arc A0 (-12.3, 29.3) -> (-12.3, 34.3) centre (-12.3, 31.8) ccw
  line L1 (-12.3, 29.3) -> (-42.3, 29.3)
  arc A1 (-42.3, 34.3) -> (-42.3, 29.3) centre (-42.3, 31.8) ccw
  line L2 (-42.3, 44.3) -> (-12.3, 44.3)
  arc A2 (-12.3, 39.3) -> (-12.3, 44.3) centre (-12.3, 41.8) ccw
  line L3 (-12.3, 39.3) -> (-42.3, 39.3)
  arc A3 (-42.3, 44.3) -> (-42.3, 39.3) centre (-42.3, 41.8) ccw
  line L4 (-42.3, 24.3) -> (-12.3, 24.3)
  arc A4 (-12.3, 19.3) -> (-12.3, 24.3) centre (-12.3, 21.8) ccw
  line L5 (-12.3, 19.3) -> (-42.3, 19.3)
  arc A5 (-42.3, 24.3) -> (-42.3, 19.3) centre (-42.3, 21.8) ccw
  line L6 (-42.3, 74.3) -> (-12.3, 74.3)
  arc A6 (-12.3, 69.3) -> (-12.3, 74.3) centre (-12.3, 71.8) ccw
  line L7 (-12.3, 69.3) -> (-42.3, 69.3)
  arc A7 (-42.3, 74.3) -> (-42.3, 69.3) centre (-42.3, 71.8) ccw
  line L8 (45.7, 29.3) -> (15.7, 29.3)
  arc A8 (15.7, 34.3) -> (15.7, 29.3) centre (15.7, 31.8) ccw
  line L9 (15.7, 34.3) -> (45.7, 34.3)
  arc A9 (45.7, 29.3) -> (45.7, 34.3) centre (45.7, 31.8) ccw
  circle A10 centre (-29, -58) radius 2
  circle A11 centre (-29, -67) radius 2
  circle A12 centre (-20, -58) radius 2
  circle A13 centre (-20, -67) radius 2
  arc A14 (-34.5896, -90.2209) -> (-14.4104, -90.2209) centre (-24.5, -62.5) ccw
  arc A15 (-32.5375, -84.5828) -> (-34.5896, -90.2209) centre (-33.5635, -87.4019) ccw
  arc A16 (-32.5375, -84.5828) -> (-16.4625, -84.5828) centre (-24.5, -62.5) ccw
  arc A17 (-14.4104, -90.2209) -> (-16.4625, -84.5828) centre (-15.4365, -87.4019) ccw
  arc A18 (-9.2972, -47.2972) -> (-18.9354, -41.7326) centre (-24.5, -62.5) ccw
  arc A19 (-13.5398, -51.5398) -> (-9.2972, -47.2972) centre (-11.4185, -49.4185) ccw
  arc A20 (-13.5398, -51.5398) -> (-20.4883, -47.5281) centre (-24.5, -62.5) ccw
  arc A21 (-18.9354, -41.7326) -> (-20.4883, -47.5281) centre (-19.7118, -44.6304) ccw
  arc A22 (-45.2674, -56.9354) -> (-45.2674, -68.0646) centre (-24.5, -62.5) ccw
  arc A23 (-39.4719, -58.4883) -> (-45.2674, -56.9354) centre (-42.3696, -57.7118) ccw
  arc A24 (-39.4719, -58.4883) -> (-39.4719, -66.5117) centre (-24.5, -62.5) ccw
  arc A25 (-45.2674, -68.0646) -> (-39.4719, -66.5117) centre (-42.3696, -67.2882) ccw
  arc A26 (-39.7028, -77.7028) -> (-30.0646, -83.2674) centre (-24.5, -62.5) ccw
  arc A27 (-35.4602, -73.4602) -> (-39.7028, -77.7028) centre (-37.5815, -75.5815) ccw
  arc A28 (-35.4602, -73.4602) -> (-28.5117, -77.4719) centre (-24.5, -62.5) ccw
  arc A29 (-30.0646, -83.2674) -> (-28.5117, -77.4719) centre (-29.2882, -80.3696) ccw
  arc A30 (-14.4104, -34.7791) -> (-34.5896, -34.7791) centre (-24.5, -62.5) ccw
  arc A31 (-16.4625, -40.4172) -> (-14.4104, -34.7791) centre (-15.4365, -37.5981) ccw
  arc A32 (-16.4625, -40.4172) -> (-32.5375, -40.4172) centre (-24.5, -62.5) ccw
  arc A33 (-34.5896, -34.7791) -> (-32.5375, -40.4172) centre (-33.5635, -37.5981) ccw
  arc A34 (-53.5518, -67.6226) -> (-43.4622, -85.0983) centre (-24.5, -62.5) ccw
  arc A35 (-47.643, -66.5807) -> (-53.5518, -67.6226) centre (-50.5974, -67.1017) ccw
  arc A36 (-47.643, -66.5807) -> (-39.6055, -80.502) centre (-24.5, -62.5) ccw
  arc A37 (-43.4622, -85.0983) -> (-39.6055, -80.502) centre (-41.5339, -82.8002) ccw
  arc A38 (-5.5378, -85.0983) -> (4.5518, -67.6226) centre (-24.5, -62.5) ccw
  arc A39 (-9.3945, -80.502) -> (-5.5378, -85.0983) centre (-7.4661, -82.8002) ccw
  arc A40 (-9.3945, -80.502) -> (-1.357, -66.5807) centre (-24.5, -62.5) ccw
  arc A41 (4.5518, -67.6226) -> (-1.357, -66.5807) centre (1.5974, -67.1017) ccw
  arc A42 (-3.7326, -68.0646) -> (-3.7326, -56.9354) centre (-24.5, -62.5) ccw
  arc A43 (-9.5281, -66.5117) -> (-3.7326, -68.0646) centre (-6.6304, -67.2882) ccw
  arc A44 (-9.5281, -66.5117) -> (-9.5281, -58.4883) centre (-24.5, -62.5) ccw
  arc A45 (-3.7326, -56.9354) -> (-9.5281, -58.4883) centre (-6.6304, -57.7118) ccw
  arc A46 (-30.0646, -41.7326) -> (-39.7028, -47.2972) centre (-24.5, -62.5) ccw
  arc A47 (-28.5117, -47.5281) -> (-30.0646, -41.7326) centre (-29.2882, -44.6304) ccw
  arc A48 (-28.5117, -47.5281) -> (-35.4602, -51.5398) centre (-24.5, -62.5) ccw
  arc A49 (-39.7028, -47.2972) -> (-35.4602, -51.5398) centre (-37.5815, -49.4185) ccw
  arc A50 (-18.9354, -83.2674) -> (-9.2972, -77.7028) centre (-24.5, -62.5) ccw
  arc A51 (-20.4883, -77.4719) -> (-18.9354, -83.2674) centre (-19.7118, -80.3696) ccw
  arc A52 (-20.4883, -77.4719) -> (-13.5398, -73.4602) centre (-24.5, -62.5) ccw
  arc A53 (-9.2972, -77.7028) -> (-13.5398, -73.4602) centre (-11.4185, -75.5815) ccw
  arc A54 (4.5518, -57.3774) -> (-5.5378, -39.9017) centre (-24.5, -62.5) ccw
  arc A55 (-1.357, -58.4193) -> (4.5518, -57.3774) centre (1.5974, -57.8983) ccw
  arc A56 (-1.357, -58.4193) -> (-9.3945, -44.498) centre (-24.5, -62.5) ccw
  arc A57 (-5.5378, -39.9017) -> (-9.3945, -44.498) centre (-7.4661, -42.1998) ccw
  arc A58 (-43.4622, -39.9017) -> (-53.5518, -57.3774) centre (-24.5, -62.5) ccw
  arc A59 (-39.6055, -44.498) -> (-43.4622, -39.9017) centre (-41.5339, -42.1998) ccw
  arc A60 (-39.6055, -44.498) -> (-47.643, -58.4193) centre (-24.5, -62.5) ccw
  arc A61 (-53.5518, -57.3774) -> (-47.643, -58.4193) centre (-50.5974, -57.8983) ccw
  line L10 (60, 96.1) -> (-60, 96.1)
  line L11 (-60, 96.1) -> (-60, -110.5)
  line L12 (-60, -110.5) -> (60, -110.5)
  line L13 (60, -110.5) -> (60, 96.1)
  line L14 (60, 96.1) -> (-60, 96.1)
  line L15 (60, 94.1) -> (-60, 94.1)
  dimension "d115" = -2
extrude "Extrude18" add sketch "Sketch15" along normal blind 16.5 contours L10 L11 L13 L14 L15 bodies 1
equation "d38 = ( 3 / 2 ) * 1 mm + 4 mm"
equation "d39 = ( 7 / 2 ) * 1 mm + 3 mm"
equation "d40 = ( 7 / 2 ) * 1 mm + 12.5 mm"
equation "d62 = ( 360 / 18 / 2 ) * 1 deg"
equation "d72 = 35 mm - 5 mm"
equation "d85 = -23 mm - 35 mm"
equation "d116 = 18.5 mm - 2 mm"
